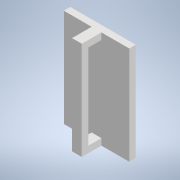
# Autodesk Inventor part: Клемники винтовые
Saved by Autodesk Inventor 2021.2 (Build 252289000, 289)
## iProperties
Created: 2021-10-12
Part Number: Клемники винтовые
Material: Типовые
Document SubType Name: Modeling
Designer: Surflay
Density: 1 g/cm^3
Appearance: По умолчанию
Categories: <MemberInstance><Categories><Category DisplayName="" Mnemonic="CABLEANDHARNESS" InternalName="e4a7e005-5e42-4d16-b293-125e7f0d0512"><Category DisplayName="" Mnemonic="CONNECTORS" InternalName="6f634eba-a678-4820-a31d-2c2d5ee6728e"><CategoryParameter DisplayName="" Mnemonic="REFDES" InternalName="c3740e8c-60ab-4d5d-8584-52b73222f2f0"/><Category DisplayName="" Mnemonic="DISCRETEWIRE" InternalName="9a3407de-09b2-4cdb-8c40-9708d5144a28"/></Category></Category></Categories><FamilyTemplate><FamilyTemplateParameters></FamilyTemplateParameters></FamilyTemplate><CategoryParameterMap><ParamToTemplateMap><ParamToTemplate CategoryParameter="//CategoryParameter[@InternalName='c3740e8c-60ab-4d5d-8584-52b73222f2f0']" ConstantValue=""/></ParamToTemplateMap></CategoryParameterMap></MemberInstance>
Author: Surflay
Autodesk Inventor part; units mm, degrees
ref_plane "YZ Plane" through (0, 0, 0) normal (1, 0, 0) x (0, 1, 0)
ref_plane "XZ Plane" through (0, 0, 0) normal (0, 1, 0) x (-1, 0, 0)
ref_plane "XY Plane" through (0, 0, 0) normal (0, 0, 1) x (1, 0, 0)
sketch "Эскиз1" plane through (0, 0, 0) normal (0, 0, 1) x (1, 0, 0)
  line L0 (29.925, -19.7625) -> (39.925, -19.7625)
  line L1 (39.925, -19.7625) -> (39.925, -34.7625)
  line L2 (39.925, -34.7625) -> (29.925, -34.7625)
  line L3 (29.925, -34.7625) -> (29.925, -19.7625)
  point P0 (0, 0)
  dimension "d0" = 15
  dimension "d1" = 10
  constraints: 8 end point, 2 parallel, 1 horizontal, 1 perpendicular
  measures "d0" distance between parallel lines of L2 L0
  measures "d1" distance between parallel lines of L3 L1
extrude "Выдавливание1" add sketch "Эскиз1" along normal blind 5
sketch "Эскиз2" plane through (29.925, -34.7625, 0) normal (0, -1, 0) x (1, 0, 0)
  line L0 (0, 0) -> (0, 5) projected
  line L1 (0, 1) -> (4.25, 1)
  line L2 (4.25, 1) -> (4.25, 4)
  line L3 (4.25, 4) -> (5.75, 4)
  line L4 (5.75, 4) -> (5.75, 1)
  line L5 (5.75, 1) -> (10, 1)
  line L6 (10, 0) -> (10, 5) projected
  line L7 (0, 5) -> (10, 5) projected
  line L8 (0, 0) -> (10, 0) projected
  point P0 (-29.925, 0)
  dimension "d4" = 1.5
  dimension "d5" = 4.25
  dimension "d6" = 10
  dimension "d7" = 1
  dimension "d8" = 1
  constraints: 10 end point, 4 point on line, 3 perpendicular, 1 horizontal
  measures "d4" distance of L2.end L3.end
  measures "d5" distance between parallel lines of L6 L4
  measures "d6" distance between parallel lines of L0 L6
  measures "d7" distance between parallel lines of L7 L3
  measures "d8" distance between parallel lines of L8 L1
extrude "Выдавливание2" cut sketch "Эскиз2" against normal through all contours L0 L1 L2 L3 L4 L5 L6 L8 keep common part
sketch "Эскиз3" plane through (35.675, -34.7625, 4) normal (1, 0, 0) x (0, 0, -1)
  line L0 (3, 15) -> (0, 15) projected
  line L1 (0, 0) -> (0, 15) projected
  line L2 (0, 0) -> (3, 0) projected
  line L3 (3, 0) -> (3, 15) projected
  line L4 (3, 0) -> (3, 15) projected
  line L5 (3, 1) -> (1, 1)
  line L6 (1, 1) -> (1, 14)
  line L7 (1, 14) -> (3, 14)
  line L8 (3, 14) -> (3, 1)
  point P0 (4, 34.7625)
  point P1 (3, 1)
  dimension "d11" = 1
  dimension "d12" = 1
  dimension "d13" = 1
  constraints: 8 end point, 2 parallel, 1 horizontal, 1 perpendicular, 1 point on line
  measures "d11" distance between parallel lines of L1 L6
  measures "d12" distance between parallel lines of L0 L7
  measures "d13" distance between parallel lines of L2 L5
extrude "Выдавливание3" cut sketch "Эскиз3" against normal through all contours L3 L5 L6 L7
equation "\"d5\" = -0.5 * d4 + 0.5 * d6"
